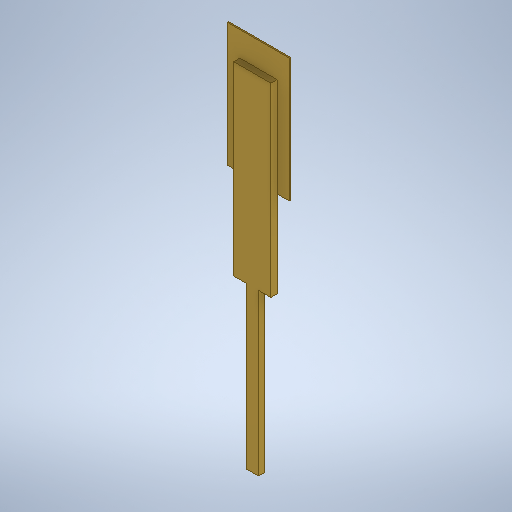
# Autodesk Inventor part: pin
Saved by Autodesk Inventor 2025 (Build 290162000, 162)
## iProperties
Created: 2025-09-08
Part Number: pin
Material: Gold
Document SubType Name: Modeling
Designer: jirne
Density: 19.3 g/cm^3
Appearance: Metal 1600F Hot
Author: jirne
Autodesk Inventor part; units mm, degrees
ref_plane "YZ Plane" through (0, 0, 0) normal (1, 0, 0) x (0, 1, 0)
ref_plane "XZ Plane" through (0, 0, 0) normal (0, 1, 0) x (-1, 0, 0)
ref_plane "XY Plane" through (0, 0, 0) normal (0, 0, 1) x (1, 0, 0)
sketch "Sketch1" plane through (0, 0, 0) normal (0, 1, 0) x (-1, 0, 0)
  line L0 (0, 0) -> (-1.27, 0)
  line L1 (-1.27, 0) -> (-1.27, 2.54)
  line L2 (-1.27, 2.54) -> (0, 2.54)
  line L3 (0, 2.54) -> (0, 0)
  dimension "d0" = 1.27
  dimension "d1" = 2.54
  constraints: 8 end point, 2 parallel, 1 horizontal, 1 perpendicular
  measures "d0" distance of L1.end L2.end
  measures "d1" distance of L0.end L1.end
extrude "Extrusion1" add sketch "Sketch1" along normal blind 0.0254
sketch "Sketch2" plane through (0, 0, 0) normal (0, -1, 0) x (1, 0, 0)
  line L0 (0, 0) -> (0, 2.54) projected
  line L1 (0.254, 2.032) -> (0.254, -1.778)
  line L2 (0.254, -1.778) -> (0.508, -1.778)
  line L3 (0.508, -1.778) -> (0.508, -5.08)
  line L4 (0.508, -5.08) -> (0.762, -5.08)
  line L5 (0.762, -5.08) -> (0.762, -1.778)
  line L6 (0.762, -1.778) -> (1.016, -1.778)
  line L7 (1.016, -1.778) -> (1.016, 2.032)
  line L8 (1.016, 2.032) -> (0.254, 2.032)
  line L9 (0, 2.54) -> (1.27, 2.54) projected
  point P0 (0.254, 2.032)
  dimension "d4" = 0.762
  dimension "d5" = 3.81
  dimension "d6" = 3.302
  dimension "d7" = 0.254
  dimension "d8" = 0.254
  dimension "d9" = 0.508
  constraints: 16 end point, 6 perpendicular, 2 point on line, 1 collinear, 1 parallel
  measures "d4" distance of L7.end L1.start
  measures "d5" distance from line of L6.end L8
  measures "d6" distance of L2.end L3.end
  measures "d7" distance of L3.end L4.end
  measures "d8" distance from line of L0 point (0.254, 2.032)
  measures "d9" distance from line of L9 point (0.254, 2.032)
extrude "Extrusion2" add sketch "Sketch2" along normal blind 0.127
body "Solid1"
